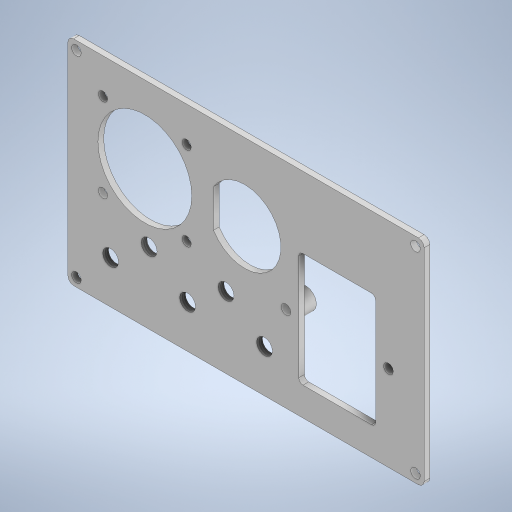
# Autodesk Inventor part: LI0011-IO SHIELD
Saved by Autodesk Inventor 2023 (Build 270158000, 158)
## iProperties
Created: 2023-04-24
Part Number: LI0011-IO SHIELD
Material: Generic
Document SubType Name: Modeling
Designer: Louis
Density: 1 g/cm^3
Appearance: Default
Author: Louis
Autodesk Inventor part; units mm, degrees
ref_plane "YZ Plane" through (0, 0, 0) normal (1, 0, 0) x (0, 1, 0)
ref_plane "XZ Plane" through (0, 0, 0) normal (0, 1, 0) x (-1, 0, 0)
ref_plane "XY Plane" through (0, 0, 0) normal (0, 0, 1) x (1, 0, 0)
sketch "Sketch1" plane through (0, 0, 0) normal (0, 0, 1) x (1, 0, 0)
  line L0 (-62.5, 37.5) -> (62.5, 37.5)
  line L1 (62.5, 37.5) -> (62.5, -37.5)
  line L2 (62.5, -37.5) -> (-62.5, -37.5)
  line L3 (-62.5, -37.5) -> (-62.5, 37.5)
  point P0 (0, 0)
  point P1 (-62.5, 0)
  point P2 (0, 37.5)
  dimension "d0" = 125
  dimension "d1" = 75
  constraints: 8 end point, 2 midpoint, 2 parallel, 1 horizontal, 1 horizontal alignment, 1 perpendicular, 1 vertical alignment
  measures "d0" distance of L0.start L0.end
  measures "d1" distance of L2.end L0.start
extrude "Extrusion1" add sketch "Sketch1" along normal blind 2
sketch "Sketch2" plane through (0, 0, 2) normal (0, 0, 1) x (1, 0, 0)
  line L0 (-62.5, -37.5) -> (62.5, -37.5) projected
  line L1 (62.5, -37.5) -> (62.5, 37.5) projected
  line L2 (62.5, 37.5) -> (-62.5, 37.5) projected
  line L3 (-62.5, 37.5) -> (-62.5, -37.5) projected
  line L4 (-59.5, 34.5) -> (59.5, 34.5)
  line L5 (59.5, 34.5) -> (59.5, -34.5)
  line L6 (59.5, -34.5) -> (-59.5, -34.5)
  line L7 (-59.5, -34.5) -> (-59.5, 34.5)
  point P0 (0, 0)
  dimension "d4" = 3
  constraints: 8 end point, 4 coincident, 3 other
  measures "d4" distance between parallel lines of L2 L4
hole "Hole1" at (-59.5, 34.5, 2) at (59.5, 34.5, 2) at (-59.5, -34.5, 2) at (59.5, -34.5, 2) direction (0, 0, -1) diameter 3.4 end through all clearance for "Oval Head Machine Screw" size "M3" standard "Ansi Metric M Profile"
fillet "Fillet1" radius 2 4 edges at (-62.5, 37.5, 1) (-62.5, -37.5, 1) (62.5, -37.5, 1) (62.5, 37.5, 1)
sketch "Sketch3" plane through (0, 0, 2) normal (0, 0, 1) x (1, 0, 0)
  line L0 (18.5, 12.5) -> (45.5, 12.5)
  line L1 (45.5, 12.5) -> (45.5, -27.5)
  line L2 (45.5, -27.5) -> (18.5, -27.5)
  line L3 (18.5, -27.5) -> (18.5, 12.5)
  line L4 (62.5, -35.5) -> (62.5, 35.5) projected
  line L5 (60.5, 37.5) -> (-60.5, 37.5) projected
  point P0 (0, 0)
  dimension "d13" = 27
  dimension "d14" = 40
  dimension "d16" = 17
  dimension "d73" = 25
  constraints: 8 end point, 2 parallel, 1 horizontal, 1 perpendicular
  measures "d13" distance of L0.start L0.end
  measures "d14" distance of L0.end L1.end
  measures "d16" distance between parallel lines of L4 L1
  measures "d73" distance between parallel lines of L5 L0
extrude "Extrusion2" cut sketch "Sketch3" against normal through all
fillet "Fillet2" radius 1.5 4 edges at (18.5, -27.5, 1) (18.5, 12.5, 1) (45.5, 12.5, 1) (45.5, -27.5, 1)
sketch "Sketch4" plane through (0, 0, 2) normal (0, 0, 1) x (1, 0, 0)
  line L0 (44, 12.5) -> (20, 12.5) projected
  line L1 (44, -27.5) -> (20, -27.5) projected
  line L2 (18.5, -26) -> (18.5, 11) projected
  line L3 (20, 12.5) -> (44, 12.5) projected
  line L4 (45.5, 11) -> (45.5, -26) projected
  line L5 (14.0041, -17.1435) -> (14.0041, 2.1435)
  line L6 (49.9959, 2.1435) -> (49.9959, -17.1435)
  line L7 (32, 12.5) -> (32, -27.5)
  point P0 (0, 0)
  point P1 (14.0041, -7.5)
  point P2 (49.9959, -7.5)
  point P3 (18.5, -7.5)
  point P4 (45.5, -7.5)
  dimension "d21" = 35.9918
  constraints: 6 end point, 6 midpoint, 2 horizontal alignment, 2 parallel, 1 other
  measures "d21" distance between parallel lines of L6 L5
hole "Hole2" at (14.0041, -7.5, 2) at (49.9959, -7.5, 2) direction (0, 0, -1) diameter 3.4 depth 6 tip angle 118 clearance for "Oval Head Machine Screw" size "M3" standard "Ansi Metric M Profile"
sketch "Sketch6" plane through (0, 0, 2) normal (0, 0, 1) x (1, 0, 0)
  circle A0 centre (-0.5, 10.5) radius 12.75
  line L0 (-11.4, 17.1146) -> (-11.4, 3.8854)
  line L1 (-62.5, 35.5) -> (-62.5, -35.5) projected
  line L2 (60.5, 37.5) -> (-60.5, 37.5) projected
  point P0 (0, 0)
  dimension "d35" = 25.5
  dimension "d36" = 10.9
  dimension "d74" = 62
  dimension "d75" = 27
  constraints: 2 end point, 2 point on circle, 1 centre point, 1 vertical
  measures "d35" diameter of A0
  measures "d36" distance from line of A0.centre L0
  measures "d74" distance from line of L1 A0.centre
  measures "d75" distance from line of A0.centre L2
extrude "Extrusion4" cut sketch "Sketch6" against normal blind 10 contours A0 L0 picked at (-2.2841, 10.5)
sketch "Sketch7" plane through (0, 0, 2) normal (0, 0, 1) x (1, 0, 0)
  line L0 (-47.5, -22.5) -> (6.5, -22.5)
  line L1 (-62.5, 35.5) -> (-62.5, -35.5) projected
  line L2 (-60.5, -37.5) -> (60.5, -37.5) projected
  line L3 (-34, -12.5) -> (-7, -12.5)
  point P0 (0, 0)
  point P1 (-20.5, -22.5)
  point P2 (-20.5, -12.5)
  dimension "d40" = 54
  dimension "d43" = 15
  dimension "d56" = 15
  dimension "d57" = 10
  dimension "d58" = 27
  constraints: 4 coincident, 4 end point, 2 horizontal, 2 midpoint, 1 vertical alignment
  measures "d40" distance of point (6.5, -22.5) point (-47.5, -22.5)
  measures "d43" distance from line of L1 L0.start
  measures "d56" distance between parallel lines of L2 L0
  measures "d57" distance between parallel lines of L0 L3
  measures "d58" distance of L3.start L3.end
hole "Hole3" at (-47.5, -22.5, 2) at (6.5, -22.5, 2) at (-20.5, -22.5, 2) at (-34, -12.5, 2) at (-7, -12.5, 2) direction (0, 0, -1) diameter 5.588 end through all thread size "1/4-36 UNS" class "2B" standard "ANSI Unified Screw Threads"
sketch "Sketch8" plane through (0, 0, 0) normal (0, 0, -1) x (-1, 0, 0)
  circle A0 centre (-49.9959, -7.5) radius 1.7 projected
  circle A1 centre (-14.0041, -7.5) radius 1.7 projected
  circle A2 centre (-49.9959, -7.5) radius 3.7
  circle A3 centre (-14.0041, -7.5) radius 3.7
  point P0 (0, 0)
  dimension "d52" = 2
  dimension "d53" = 2
  constraints: 2 centre point
  measures "d52" radial gap between concentric circles of A0 A2
  measures "d53" radial gap between concentric circles of A1 A3
extrude "Extrusion5" add sketch "Sketch8" along normal blind 5
sketch "Sketch9" plane through (0, 0, 2) normal (0, 0, 1) x (1, 0, 0)
  circle A0 centre (-35.5, 10.5) radius 16.47
  line L0 (60.5, 37.5) -> (-60.5, 37.5) projected
  line L1 (-62.5, 35.5) -> (-62.5, -35.5) projected
  line L2 (-50.18, 25.18) -> (-20.82, 25.18)
  line L3 (-20.82, 25.18) -> (-20.82, -4.18)
  line L4 (-20.82, -4.18) -> (-50.18, -4.18)
  line L5 (-50.18, -4.18) -> (-50.18, 25.18)
  point P0 (0, 0)
  point P1 (-20.82, 10.5)
  point P2 (-35.5, 25.18)
  dimension "d59" = 32.94
  dimension "d60" = 27
  dimension "d61" = 27
  dimension "d62" = 29.36
  dimension "d63" = 29.36
  constraints: 8 end point, 4 coincident, 2 midpoint, 2 parallel, 1 centre point, 1 horizontal, 1 horizontal alignment, 1 perpendicular, 1 vertical alignment
  measures "d59" diameter of A0
  measures "d60" distance from line of L0 A0.centre
  measures "d61" distance from line of L1 A0.centre
  measures "d62" distance of L2.start L2.end
  measures "d63" distance of L2.end L3.end
extrude "Extrusion6" cut sketch "Sketch9" against normal blind 10 contours A0 L3 | L3 A0 L4 L5 L2 | L2 A0 | A0 L4 | L5 A0
hole "Hole4" at (-50.18, 25.18, 2) at (-20.82, 25.18, 2) at (-50.18, -4.18, 2) at (-20.82, -4.18, 2) direction (0, 0, -1) diameter 3.25 end through all
body "Solid1"
